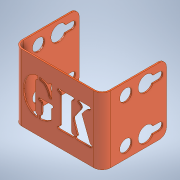
# Autodesk Inventor part: Head_GK_cloth
Saved by Autodesk Inventor 2020.4 (Build 244396000, 396)
## iProperties
Created: 2022-06-21
Part Number: Head_GK_cloth
Material: 一般
Document SubType Name: Modeling
Designer: Masato Kubotera
Density: 1 g/cm^3
Appearance: 滑らか - 淡いオレンジ
Author: Masato Kubotera
Autodesk Inventor part; units mm, degrees
ref_plane "YZ Plane" through (0, 0, 0) normal (1, 0, 0) x (0, 1, 0)
ref_plane "XZ Plane" through (0, 0, 0) normal (0, 1, 0) x (-1, 0, 0)
ref_plane "XY Plane" through (0, 0, 0) normal (0, 0, 1) x (1, 0, 0)
sketch "スケッチ1" plane through (0, 0, 0) normal (1, 0, 0) x (0, 1, 0)
  line L0 (-54.6, 19) -> (54.6, 19)
  line L1 (58.6, 15) -> (58.6, -15)
  line L2 (54.6, -19) -> (-54.6, -19)
  line L3 (-58.6, -15) -> (-58.6, 15)
  line L4 (-58.6, 19) -> (58.6, -19) construction
  line L5 (58.6, 19) -> (-58.6, -19) construction
  arc A0 (-50.9799, 10.4) -> (-50.9799, 14.6) centre (-47, 12.5) ccw
  line L6 (-54.5, 10.4) -> (-50.9799, 10.4)
  line L7 (-54.5, 14.6) -> (-50.9799, 14.6)
  arc A1 (-54.5, 14.6) -> (-54.5, 10.4) centre (-54.5, 12.5) ccw
  line L8 (-54.5, 12.5) -> (-47, 12.5) construction
  line L9 (-58.6, 0) -> (58.6, 0) construction
  line L10 (-54.5, 19) -> (-54.5, -19) construction
  line L11 (-58.6, -19) -> (58.6, 19) construction
  line L12 (-54.5, -14.6) -> (-50.9799, -14.6)
  arc A2 (-54.5, -10.4) -> (-54.5, -14.6) centre (-54.5, -12.5) ccw
  line L13 (-54.5, -10.4) -> (-50.9799, -10.4)
  arc A3 (-50.9799, -14.6) -> (-50.9799, -10.4) centre (-47, -12.5) ccw
  line L14 (-54.5, -12.5) -> (-47, -12.5) construction
  line L15 (-54.5, -19) -> (-54.5, 19) construction
  line L16 (0, 19) -> (0, -19) construction
  line L17 (58.6, 19) -> (-58.6, -19) construction
  line L18 (-58.6, 19) -> (58.6, -19) construction
  line L19 (54.5, 14.6) -> (50.9799, 14.6)
  arc A4 (54.5, 10.4) -> (54.5, 14.6) centre (54.5, 12.5) ccw
  line L20 (54.5, 10.4) -> (50.9799, 10.4)
  arc A5 (50.9799, 14.6) -> (50.9799, 10.4) centre (47, 12.5) ccw
  line L21 (54.5, 12.5) -> (47, 12.5) construction
  line L22 (58.6, 0) -> (-58.6, 0) construction
  line L23 (54.5, 19) -> (54.5, -19) construction
  arc A6 (54.5, -14.6) -> (54.5, -10.4) centre (54.5, -12.5) ccw
  line L24 (54.5, -14.6) -> (50.9799, -14.6)
  line L25 (54.5, -10.4) -> (50.9799, -10.4)
  line L26 (54.5, -12.5) -> (47, -12.5) construction
  arc A7 (50.9799, -10.4) -> (50.9799, -14.6) centre (47, -12.5) ccw
  line L27 (54.5, -19) -> (54.5, 19) construction
  line L28 (58.6, -19) -> (-58.6, 19) construction
  line L29 (-9.5939, 5.613) -> (9.5939, 5.613) construction
  line L30 (9.5939, 5.613) -> (9.5939, -5.613) construction
  line L31 (9.5939, -5.613) -> (-9.5939, -5.613) construction
  line L32 (-9.5939, -5.613) -> (-9.5939, 5.613) construction
  line L33 (-9.5939, 5.613) -> (9.5939, -5.613) construction
  line L34 (9.5939, 5.613) -> (-9.5939, -5.613) construction
  arc A8 (-54.6, 19) -> (-58.6, 15) centre (-54.6, 15) ccw
  arc A9 (-58.6, -15) -> (-54.6, -19) centre (-54.6, -15) ccw
  arc A10 (58.6, 15) -> (54.6, 19) centre (54.6, 15) ccw
  arc A11 (54.6, -19) -> (58.6, -15) centre (54.6, -15) ccw
  line L35 (-20.5, 19) -> (-20.5, -19)
  line L36 (20.5, 19) -> (20.5, -19)
  line L37 (-16.5, 19) -> (-16.5, -19) construction
  line L38 (16.5, 19) -> (16.5, -19) construction
  line L39 (-24.5, 19) -> (-24.5, -19) construction
  line L40 (24.5, 19) -> (24.5, -19) construction
  circle A12 centre (-35.5, 12.5) radius 3.5
  circle A13 centre (-35.5, -12.5) radius 3.5
  circle A14 centre (35.5, 12.5) radius 3.5
  circle A15 centre (35.5, -12.5) radius 3.5
  line L41 (-11.4757, 10.3993) -> (-11.4757, 8.7674)
  spline S0 degree 2 poles (-11.4757, 8.7674) (-12.7604, 8.4549) (-12.7604, 6.7187) knots 0 0 0 1 1 1
  line L42 (-12.7604, 6.7187) -> (-12.7604, -6.9271)
  spline S1 degree 2 poles (-12.7604, -6.9271) (-12.7604, -7.7083) (-12.5347, -8.1424) knots 0 0 0 1 1 1
  spline S2 degree 2 poles (-12.5347, -8.1424) (-12.3438, -8.4896) (-11.7361, -8.7326) knots 0 0 0 1 1 1
  line L43 (-11.7361, -8.7326) -> (-11.7361, -10.3993)
  spline S3 degree 2 poles (-11.7361, -10.3993) (-12.2049, -10.3993) (-12.9861, -10.2431) (-13.6285, -10.0347) knots 0 0 0 1 2 2 2
  spline S4 degree 2 poles (-13.6285, -10.0347) (-15.1563, -9.4965) (-17.6563, -7.3264) (-18.4549, -5.816) knots 0 0 0 1 2 2 2
  spline S5 degree 2 poles (-18.4549, -5.816) (-19.7049, -3.4722) (-19.7049, -0.2431) knots 0 0 0 1 1 1
  spline S6 degree 2 poles (-19.7049, -0.2431) (-19.7049, 2.8819) (-17.4826, 7.7083) (-15.3993, 9.0972) knots 0 0 0 1 2 2 2
  spline S7 degree 2 poles (-15.3993, 9.0972) (-14.2014, 9.8958) (-12.8299, 10.2431) knots 0 0 0 1 1 1
  spline S8 degree 2 poles (-12.8299, 10.2431) (-12.2569, 10.3993) (-11.4757, 10.3993) knots 0 0 0 1 1 1
  spline S9 degree 2 poles (-3.6632, -7.5521) (-4.2535, -8.1424) (-6.1979, -9.3576) (-7.066, -9.7049) knots 0 0 0 1 2 2 2
  spline S10 degree 2 poles (-7.066, -9.7049) (-7.8472, -10.0174) (-9.7743, -10.3993) (-10.5035, -10.3993) knots 0 0 0 1 2 2 2
  line L44 (-10.5035, -10.3993) -> (-10.5035, -8.7326)
  spline S11 degree 2 poles (-10.5035, -8.7326) (-10.0694, -8.6458) (-9.6528, -8.3507) (-9.4965, -8.0729) knots 0 0 0 1 2 2 2
  spline S12 degree 2 poles (-9.4965, -8.0729) (-9.2535, -7.6215) (-9.2535, -6.9271) knots 0 0 0 1 1 1
  line L45 (-9.2535, -6.9271) -> (-9.2535, -2.6389)
  spline S13 degree 2 poles (-9.2535, -2.6389) (-9.2535, -2.066) (-9.4792, -1.8229) knots 0 0 0 1 1 1
  spline S14 degree 2 poles (-9.4792, -1.8229) (-9.5833, -1.684) (-9.7743, -1.5972) (-10.3472, -1.4757) knots 0 0 0 1 2 2 2
  spline S15 degree 2 poles (-10.3472, -1.4757) (-11.059, -1.3021) (-11.059, -0.6597) knots 0 0 0 1 1 1
  spline S16 degree 2 poles (-11.059, -0.6597) (-11.059, -0.2778) (-10.3993, 0.1389) (-9.7569, 0.1389) knots 0 0 0 1 2 2 2
  line L46 (-9.7569, 0.1389) -> (-9.2708, 0.1389)
  line L47 (-9.2708, 0.1389) -> (-3.9063, 0.1389)
  spline S17 degree 2 poles (-3.9063, 0.1389) (-3.2465, 0.1389) (-2.7083, -0.2257) (-2.7083, -0.6771) knots 0 0 0 1 2 2 2
  spline S18 degree 2 poles (-2.7083, -0.6771) (-2.7083, -0.9549) (-2.934, -1.3194) (-3.2292, -1.5278) knots 0 0 0 1 2 2 2
  spline S19 degree 2 poles (-3.2292, -1.5278) (-3.5243, -1.7361) (-3.6632, -2.0833) (-3.6632, -2.5521) knots 0 0 0 1 2 2 2
  line L48 (-3.6632, -2.5521) -> (-3.6632, -7.5521)
  line L49 (-10.2778, 8.8021) -> (-10.2778, 10.3819)
  spline S20 degree 2 poles (-10.2778, 10.3819) (-7.8993, 10.1562) (-6.3542, 9.4965) knots 0 0 0 1 1 1
  spline S21 degree 2 poles (-6.3542, 9.4965) (-5.9028, 9.2882) (-5.6597, 9.2882) knots 0 0 0 1 1 1
  spline S22 degree 2 poles (-5.6597, 9.2882) (-5.4167, 9.2882) (-5.1736, 9.5139) (-4.7917, 10.0347) knots 0 0 0 1 2 2 2
  spline S23 degree 2 poles (-4.7917, 10.0347) (-4.5313, 10.3993) (-4.1319, 10.3993) knots 0 0 0 1 1 1
  spline S24 degree 2 poles (-4.1319, 10.3993) (-3.7153, 10.3993) (-3.3854, 9.9479) (-3.3854, 9.4097) knots 0 0 0 1 2 2 2
  line L50 (-3.3854, 9.4097) -> (-3.3854, 3.7153)
  spline S25 degree 2 poles (-3.3854, 3.7153) (-3.3854, 2.5868) (-4.2014, 2.5868) knots 0 0 0 1 1 1
  spline S26 degree 2 poles (-4.2014, 2.5868) (-4.6181, 2.5868) (-5.0174, 3.0208) (-5.191, 3.6806) knots 0 0 0 1 2 2 2
  spline S27 degree 2 poles (-5.191, 3.6806) (-5.3993, 4.4965) (-6.5451, 6.684) (-7.066, 7.309) knots 0 0 0 1 2 2 2
  spline S28 degree 2 poles (-7.066, 7.309) (-7.6736, 8.0556) (-9.1667, 8.7326) (-10.2778, 8.8021) knots 0 0 0 1 2 2 2
  line L51 (7.8299, -10) -> (1.2847, -10)
  line L52 (1.2847, -10) -> (0.9028, -10)
  spline S29 degree 2 poles (0.9028, -10) (0.3819, -10) (-0.191, -9.6007) (-0.191, -9.2361) knots 0 0 0 1 2 2 2
  spline S30 degree 2 poles (-0.191, -9.2361) (-0.191, -8.6458) (0.3993, -8.4549) knots 0 0 0 1 1 1
  spline S31 degree 2 poles (0.3993, -8.4549) (0.8854, -8.2813) (1.0417, -8.2118) (1.1285, -8.0729) knots 0 0 0 1 2 2 2
  spline S32 degree 2 poles (1.1285, -8.0729) (1.3021, -7.8472) (1.3021, -7.3264) knots 0 0 0 1 1 1
  line L53 (1.3021, -7.3264) -> (1.3021, 7.3264)
  spline S33 degree 2 poles (1.3021, 7.3264) (1.3021, 7.8472) (1.1285, 8.0729) knots 0 0 0 1 1 1
  spline S34 degree 2 poles (1.1285, 8.0729) (1.0417, 8.2118) (0.8854, 8.2812) (0.3993, 8.4375) knots 0 0 0 1 2 2 2
  spline S35 degree 2 poles (0.3993, 8.4375) (-0.191, 8.6285) (-0.191, 9.2361) knots 0 0 0 1 1 1
  spline S36 degree 2 poles (-0.191, 9.2361) (-0.191, 9.6007) (0.3819, 10) (0.9028, 10) knots 0 0 0 1 2 2 2
  line L54 (0.9028, 10) -> (1.2847, 10)
  line L55 (1.2847, 10) -> (7.8299, 10)
  line L56 (7.8299, 10) -> (8.2118, 10)
  spline S37 degree 2 poles (8.2118, 10) (8.7326, 10) (9.3056, 9.6007) (9.3056, 9.2361) knots 0 0 0 1 2 2 2
  spline S38 degree 2 poles (9.3056, 9.2361) (9.3056, 8.6285) (8.7153, 8.4375) knots 0 0 0 1 1 1
  spline S39 degree 2 poles (8.7153, 8.4375) (8.2292, 8.2812) (8.0729, 8.2118) (7.9861, 8.0729) knots 0 0 0 1 2 2 2
  spline S40 degree 2 poles (7.9861, 8.0729) (7.8125, 7.8472) (7.8125, 7.3264) knots 0 0 0 1 1 1
  line L57 (7.8125, 7.3264) -> (7.8125, -7.3264)
  spline S41 degree 2 poles (7.8125, -7.3264) (7.8125, -8.1597) (8.2465, -8.2986) knots 0 0 0 1 1 1
  line L58 (8.2465, -8.2986) -> (8.6979, -8.4549)
  spline S42 degree 2 poles (8.6979, -8.4549) (9.2535, -8.6285) (9.2535, -9.2361) knots 0 0 0 1 1 1
  spline S43 degree 2 poles (9.2535, -9.2361) (9.2535, -10) (8.2118, -10) knots 0 0 0 1 1 1
  line L59 (8.2118, -10) -> (7.8299, -10)
  line L60 (13.6285, 4.184) -> (18.0556, -7.3785)
  spline S44 degree 2 poles (18.0556, -7.3785) (18.2292, -7.8472) (18.6111, -8.3333) (18.9062, -8.4549) knots 0 0 0 1 2 2 2
  spline S45 degree 2 poles (18.9062, -8.4549) (19.2187, -8.6111) (19.3056, -8.6806) knots 0 0 0 1 1 1
  spline S46 degree 2 poles (19.3056, -8.6806) (19.5139, -8.8889) (19.5139, -9.2188) knots 0 0 0 1 1 1
  spline S47 degree 2 poles (19.5139, -9.2188) (19.5139, -10) (18.4028, -10) knots 0 0 0 1 1 1
  line L61 (18.4028, -10) -> (11.0417, -10)
  spline S48 degree 2 poles (11.0417, -10) (10.5208, -10) (9.9479, -9.566) (9.9479, -9.1493) knots 0 0 0 1 2 2 2
  spline S49 degree 2 poles (9.9479, -9.1493) (9.9479, -8.6806) (10.4861, -8.4201) knots 0 0 0 1 1 1
  spline S50 degree 2 poles (10.4861, -8.4201) (10.8333, -8.2639) (11.059, -8.0382) (11.0764, -7.8472) knots 0 0 0 1 2 2 2
  spline S51 degree 2 poles (11.0764, -7.8472) (11.0764, -7.7431) (10.9549, -7.3785) knots 0 0 0 1 1 1
  line L62 (10.9549, -7.3785) -> (9.0799, -1.7882)
  spline S52 degree 2 poles (9.0799, -1.7882) (8.8194, -1.0069) (8.8194, -0.4688) knots 0 0 0 1 1 1
  spline S53 degree 2 poles (8.8194, -0.4688) (8.8194, 0.0521) (9.2361, 0.6597) knots 0 0 0 1 1 1
  line L63 (9.2361, 0.6597) -> (12.7431, 5.5903)
  spline S54 degree 2 poles (12.7431, 5.5903) (13.2465, 6.2847) (13.2465, 7.0312) knots 0 0 0 1 1 1
  spline S55 degree 2 poles (13.2465, 7.0312) (13.2465, 7.4306) (12.8125, 8.1424) (12.4306, 8.2812) knots 0 0 0 1 2 2 2
  line L64 (12.4306, 8.2812) -> (11.9097, 8.5069)
  spline S56 degree 2 poles (11.9097, 8.5069) (11.4062, 8.7153) (11.4062, 9.2014) knots 0 0 0 1 1 1
  spline S57 degree 2 poles (11.4062, 9.2014) (11.4062, 9.5833) (11.7187, 9.8437) knots 0 0 0 1 1 1
  spline S58 degree 2 poles (11.7187, 9.8437) (11.9271, 10) (12.3958, 10) knots 0 0 0 1 1 1
  line L65 (12.3958, 10) -> (17.6042, 10)
  spline S59 degree 2 poles (17.6042, 10) (18.125, 10) (18.6979, 9.5486) (18.6979, 9.1319) knots 0 0 0 1 2 2 2
  spline S60 degree 2 poles (18.6979, 9.1319) (18.6979, 8.5243) (18.0208, 8.2465) knots 0 0 0 1 1 1
  line L66 (18.0208, 8.2465) -> (17.2396, 7.9514)
  spline S61 degree 2 poles (17.2396, 7.9514) (16.7535, 7.7778) (16.0069, 7.1528) knots 0 0 0 1 1 1
  spline S62 degree 2 poles (16.0069, 7.1528) (15.4514, 6.684) (14.6354, 5.5903) knots 0 0 0 1 1 1
  line L67 (14.6354, 5.5903) -> (13.6285, 4.184)
  point P0 (0, 0)
  point P1 (0, 5.613)
  point P2 (0, 0)
  point P3 (43.6458, 9.5001)
  point P4 (43.6458, 15.4999)
  point P5 (43.6458, -15.4999)
  point P6 (43.6458, -9.5001)
  point P7 (-43.6458, 15.4999)
  point P8 (-43.6458, 9.5001)
  point P9 (-43.6458, -9.5001)
  point P10 (-43.6458, -15.4999)
  dimension "d0" = 117.2
  dimension "d1" = 9
  dimension "d2" = 4.2
  dimension "d3" = 7.5
  dimension "d5" = 2
  dimension "d6" = 25
  dimension "d7" = 2
  dimension "d8" = 38
  dimension "d13" = 4
  dimension "d15" = 33
  dimension "d16" = 30
  dimension "d17" = 8
  dimension "d22" = 7
  dimension "d23" = 19
  constraints: 70 end point, 35 symmetric about line, 24 point on circle, 16 centre point, 10 point on line, 7 midpoint, 7 vertical, 6 tangent, 3 equal radius, 3 parallel, 43 other
  measures "d0" distance of L4.end L5.end
  measures "d1" diameter of A0
  measures "d2" diameter of A1
  measures "d3" distance of L8.start L8.end
  measures "d5" distance edge to line of A1 L3
  measures "d6" distance of L14.start L8.start
  measures "d8" distance of L5.start L4.end
  measures "d13" radius of A8
  measures "d15" distance of L38.start L37.start
  measures "d16" distance between parallel lines of L10 L39
  measures "d17" distance of L39.start L37.start
  measures "d22" diameter of A12
  measures "d23" distance of A12.centre L8.start
extrude "押し出し1" add sketch "スケッチ1" along normal blind 0.75 contours L0 L35 L2 A9 L3 A8 | L0 L36 L2 L35 | L0 A10 L1 A11 L2 L36 | L41 S0 L42 S1 S2 L43 S3 S4 S5 S6 S7 S8 | S9 S10 L44 S11 S12 L45 S13 S14 S15 S16 L46 L47 S17 S18 S19 L48 | L49 S20 S21 S22 S23 S24 L50 S25 S26 S27 S28 | L51 L52 S29 S30 S31 S32 L53 S33 S34 S35 S36 L54 L55 L56 S37 S38 S39 S40 L57 S41 L58 S42 S43 L59 | L60 S44 S45 S46 S47 L61 S48 S49 S50 S51 L62 S52 S53 L63 S54 S55 L64 S56 S57 S58 L65 S59 S60 L66 S61 S62 L67
extrude "押し出し2" cut sketch "スケッチ1" along normal through all contours L41 S0 L42 S1 S2 L43 S3 S4 S5 S6 S7 S8 | S9 S10 L44 S11 S12 L45 S13 S14 S15 S16 L46 L47 S17 S18 S19 L48 | L49 S20 S21 S22 S23 S24 L50 S25 S26 S27 S28 | L51 L52 S29 S30 S31 S32 L53 S33 S34 S35 S36 L54 L55 L56 S37 S38 S39 S40 L57 S41 L58 S42 S43 L59 | L60 S44 S45 S46 S47 L61 S48 S49 S50 S51 L62 S52 S53 L63 S54 S55 L64 S56 S57 S58 L65 S59 S60 L66 S61 S62 L67
bend part "曲げパーツ1" radius 4 angle 90 line through (0, -20.5, 19) along (0, 0, -1) centre toward (-1, 0, 0) moving side (0, -1, 0) both sides no
bend part "曲げパーツ2" radius 4 angle 90 line through (0, 20.5, 19) along (0, 0, -1) centre toward (-1, 0, 0) moving side (0, 1, 0) both sides no
equation "\"d7\" = d5"
equation "\"d18\" = 0.5 * d17"
equation "\"d20\" = 0.5 * d17"
